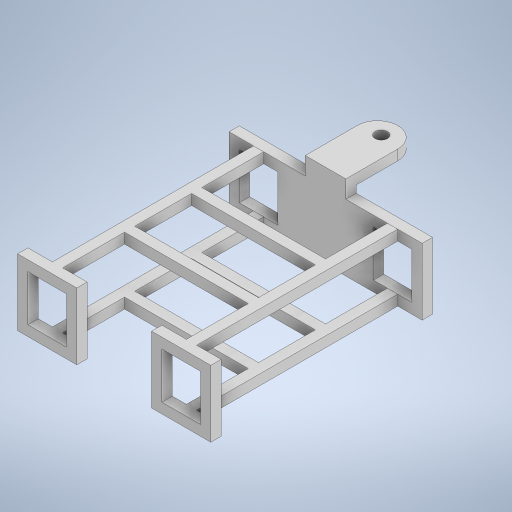
# Autodesk Inventor part: MHead
Saved by Autodesk Inventor 2024 (Build 280153000, 153)
## iProperties
Created: 2023-06-14
Part Number: MHead
Material: Generic
Document SubType Name: Modeling
Designer: vilas
Density: 1 g/cm^3
Appearance: Default
Author: vilas
Autodesk Inventor part; units mm, degrees
ref_plane "YZ Plane" through (0, 0, 0) normal (1, 0, 0) x (0, 1, 0)
sketch "Sketch1" plane through (0, 0, 0) normal (0, 0, 1) x (1, 0, 0)
  line L0 (-30, 11.15) -> (30, 11.15) construction
  line L1 (30, 11.15) -> (30, -11.15) construction
  line L2 (30, -11.15) -> (-30, -11.15) construction
  line L3 (-30, -11.15) -> (-30, 11.15) construction
  line L4 (-30, 11.15) -> (30, -11.15) construction
  line L5 (30, 11.15) -> (-30, -11.15) construction
  line L6 (-30, 11.15) -> (-35, 11.15)
  line L7 (-35, 11.15) -> (-35, 16.15)
  line L8 (-35, 16.15) -> (-30, 16.15)
  line L9 (-30, 16.15) -> (-30, 11.15)
  line L10 (30, 11.15) -> (35, 11.15)
  line L11 (35, 11.15) -> (35, 16.15)
  line L12 (35, 16.15) -> (30, 16.15)
  line L13 (30, 16.15) -> (30, 11.15)
  line L14 (30, -11.15) -> (35, -11.15)
  line L15 (35, -11.15) -> (35, -16.15)
  line L16 (35, -16.15) -> (30, -16.15)
  line L17 (30, -16.15) -> (30, -11.15)
  line L18 (-30, -11.15) -> (-35, -11.15)
  line L19 (-35, -11.15) -> (-35, -16.15)
  line L20 (-35, -16.15) -> (-30, -16.15)
  line L21 (-30, -16.15) -> (-30, -11.15)
  point P0 (0, 0)
  dimension "d0" = 60
  dimension "d1" = 22.3
  dimension "d2" = 5
  dimension "d3" = 5
  dimension "d4" = 5
  dimension "d5" = 5
  dimension "d6" = 5
  dimension "d7" = 5
  dimension "d8" = 5
  dimension "d9" = 5
  constraints: 44 end point, 10 parallel, 5 horizontal, 5 perpendicular, 2 midpoint
  measures "d0" distance of L1.end L2.end
  measures "d1" distance of L0.end L1.end
  measures "d2" distance of L7.end L8.end
  measures "d3" distance of L6.end L7.end
  measures "d4" distance of L12.end L11.end
  measures "d5" distance of L11.end L10.end
  measures "d6" distance of L15.end L16.end
  measures "d7" distance of L14.end L15.end
  measures "d8" distance of L20.end L19.end
  measures "d9" distance of L19.end L18.end
extrude "Extrusion1" add sketch "Sketch1" along normal mid plane 97.524
ref_plane "Work Plane1" through (0, 0, 48.762) normal (0, 0, 1) x (1, 0, 0)
sketch "Sketch2" plane through (0, 0, 48.762) normal (0, 0, 1) x (1, 0, 0)
  line L0 (0, 0) -> (-32.5, 0) construction
  line L1 (0, 0) -> (32.5, 0) construction
  line L2 (-46.85, 16.15) -> (-18.15, 16.15)
  line L3 (-18.15, 16.15) -> (-18.15, -16.15)
  line L4 (-18.15, -16.15) -> (-46.85, -16.15)
  line L5 (-46.85, -16.15) -> (-46.85, 16.15)
  line L6 (-46.85, 16.15) -> (-18.15, -16.15) construction
  line L7 (-18.15, 16.15) -> (-46.85, -16.15) construction
  line L8 (18.15, 16.15) -> (46.85, 16.15)
  line L9 (46.85, 16.15) -> (46.85, -16.15)
  line L10 (46.85, -16.15) -> (18.15, -16.15)
  line L11 (18.15, -16.15) -> (18.15, 16.15)
  line L12 (18.15, 16.15) -> (46.85, -16.15) construction
  line L13 (46.85, 16.15) -> (18.15, -16.15) construction
  line L14 (-23.15, 11.15) -> (-41.85, 11.15)
  line L15 (-41.85, 11.15) -> (-41.85, -11.15)
  line L16 (-41.85, -11.15) -> (-23.15, -11.15)
  line L17 (-23.15, -11.15) -> (-23.15, 11.15)
  line L18 (41.85, 11.15) -> (23.15, 11.15)
  line L19 (23.15, 11.15) -> (23.15, -11.15)
  line L20 (23.15, -11.15) -> (41.85, -11.15)
  line L21 (41.85, -11.15) -> (41.85, 11.15)
  dimension "d13" = 32.5
  dimension "d14" = 32.5
  dimension "d15" = 28.7
  dimension "d16" = 32.3
  dimension "d17" = 28.7
  dimension "d18" = 32.3
  dimension "d19" = 5
  dimension "d20" = 5
  constraints: 44 end point, 8 parallel, 4 horizontal, 4 midpoint, 4 perpendicular, 6 other
  measures "d13" distance of L0.start L0.end
  measures "d14" distance of L0.start L1.end
  measures "d15" distance of L3.end L4.end
  measures "d16" distance of L2.end L3.end
  measures "d17" distance of L9.end L10.end
  measures "d18" distance of L8.end L9.end
  measures "d19" distance between parallel lines of L2 L14
  measures "d20" distance between parallel lines of L8 L18
extrude "Extrusion2" add sketch "Sketch2" along normal blind 5
ref_plane "Work Plane2" through (0, 0, -48.771) normal (0, 0, 1) x (1, 0, 0)
sketch "Sketch4" plane through (0, 0, 0) normal (1, 0, 0) x (0, 1, 0)
  line L0 (11.15, -48.762) -> (11.15, 48.762) projected
  line L1 (11.15, 18.754) -> (16.15, 18.754)
  line L2 (16.15, 18.754) -> (16.15, 13.754)
  line L3 (16.15, 13.754) -> (11.15, 13.754)
  line L4 (11.15, 13.754) -> (11.15, 18.754)
  line L5 (-16.15, 48.762) -> (16.15, 48.762) projected
  line L6 (11.15, -13.754) -> (16.15, -13.754)
  line L7 (16.15, -13.754) -> (16.15, -18.754)
  line L8 (16.15, -18.754) -> (11.15, -18.754)
  line L9 (11.15, -18.754) -> (11.15, -13.754)
  line L10 (16.15, -48.762) -> (11.15, -48.762) projected
  line L11 (-11.15, 48.762) -> (-11.15, -48.762) projected
  line L12 (-11.15, 18.754) -> (-16.15, 18.754)
  line L13 (-16.15, 18.754) -> (-16.15, 13.754)
  line L14 (-16.15, 13.754) -> (-11.15, 13.754)
  line L15 (-11.15, 13.754) -> (-11.15, 18.754)
  line L16 (-11.15, -18.754) -> (-16.15, -18.754)
  line L17 (-16.15, -18.754) -> (-16.15, -13.754)
  line L18 (-16.15, -13.754) -> (-11.15, -13.754)
  line L19 (-11.15, -13.754) -> (-11.15, -18.754)
  line L20 (-11.15, -48.762) -> (-16.15, -48.762) projected
  point P0 (0, 0)
  dimension "d30" = 5
  dimension "d31" = 5
  dimension "d32" = 30.008
  dimension "d33" = 5
  dimension "d34" = 5
  dimension "d35" = 30.008
  dimension "d36" = 5
  dimension "d37" = 5
  dimension "d38" = 5
  dimension "d39" = 5
  dimension "d40" = 30.008
  dimension "d41" = 30.008
  constraints: 32 end point, 8 parallel, 4 horizontal, 4 perpendicular, 4 point on line
  measures "d30" distance of L2.end L3.end
  measures "d31" distance of L1.end L2.end
  measures "d32" distance between parallel lines of L1 L5
  measures "d33" distance of L7.end L8.end
  measures "d34" distance of L6.end L7.end
  measures "d35" distance between parallel lines of L8 L10
  measures "d36" distance of L14.end L13.end
  measures "d37" distance of L13.end L12.end
  measures "d38" distance of L17.end L18.end
  measures "d39" distance of L16.end L17.end
  measures "d40" distance between parallel lines of L16 L20
  measures "d41" distance between parallel lines of L12 L5
extrude "Extrusion4" add sketch "Sketch4" along normal mid plane 60
sketch "Sketch7" plane through (0, 0, -48.771) normal (0, 0, 1) x (1, 0, 0)
  line L0 (-46.85, -16.15) -> (-18.15, -16.15) projected
  line L1 (46.85, 16.15) -> (-46.85, 16.15)
  line L2 (-46.85, 16.15) -> (-46.85, -16.15)
  line L3 (-46.85, -16.15) -> (46.85, -16.15)
  line L4 (46.85, -16.15) -> (46.85, 16.15)
  line L5 (46.85, 16.15) -> (-46.85, -16.15) construction
  line L6 (-46.85, 16.15) -> (46.85, -16.15) construction
  line L7 (0, 0) -> (32.5, 0) construction
  line L8 (0, 0) -> (-32.5, 0) construction
  line L9 (41.85, -11.15) -> (23.15, -11.15) projected
  line L10 (23.15, 11.15) -> (41.85, 11.15)
  line L11 (41.85, 11.15) -> (41.85, -11.15)
  line L12 (41.85, -11.15) -> (23.15, -11.15)
  line L13 (23.15, -11.15) -> (23.15, 11.15)
  line L14 (23.15, 11.15) -> (41.85, -11.15) construction
  line L15 (41.85, 11.15) -> (23.15, -11.15) construction
  line L16 (-41.85, -11.15) -> (-41.85, 11.15) projected
  line L17 (-23.15, 11.15) -> (-41.85, 11.15)
  line L18 (-41.85, 11.15) -> (-41.85, -11.15)
  line L19 (-41.85, -11.15) -> (-23.15, -11.15)
  line L20 (-23.15, -11.15) -> (-23.15, 11.15)
  line L21 (-23.15, 11.15) -> (-41.85, -11.15) construction
  line L22 (-41.85, 11.15) -> (-23.15, -11.15) construction
  line L23 (0, 0) -> (0, 24.693) construction
  line L24 (0, 24.693) -> (9.85, 24.693) construction
  line L25 (9.85, 24.693) -> (-9.85, 24.693)
  line L26 (-9.85, 24.693) -> (-9.85, 16.15)
  line L27 (-9.85, 16.15) -> (9.85, 16.15)
  line L28 (9.85, 16.15) -> (9.85, 24.693)
  dimension "d61" = 32.5
  dimension "d62" = 32.5
  dimension "d63" = 24.693
  dimension "d64" = 9.85
  dimension "d65" = 19.7
  constraints: 52 end point, 8 parallel, 6 horizontal, 6 midpoint, 5 perpendicular, 1 point on line, 1 vertical
  measures "d61" distance of L7.start L7.end
  measures "d62" distance of L7.start L8.end
  measures "d63" distance of L7.start L23.end
  measures "d64" distance of L23.end L24.end
  measures "d65" distance of L27.end L26.end
extrude "Extrusion7" add sketch "Sketch7" against normal blind 5
sketch "Sketch8" plane through (0, 0, -53.771) normal (0, 0, -1) x (-1, 0, 0)
  line L0 (9.85, 24.693) -> (-9.85, 24.693) projected
  line L1 (9.85, 16.15) -> (9.85, 24.693) projected
  line L2 (-9.85, 24.693) -> (9.85, 24.693)
  line L3 (9.85, 24.693) -> (9.85, 19.693)
  line L4 (9.85, 19.693) -> (-9.85, 19.693)
  line L5 (-9.85, 19.693) -> (-9.85, 24.693)
  point P0 (0, 0)
  dimension "d68" = 5
  constraints: 8 end point, 2 parallel, 1 horizontal, 1 perpendicular, 1 point on line
  measures "d68" distance of L2.end L3.end
extrude "Extrusion8" add sketch "Sketch8" along normal blind 30
fillet "Fillet2" radius 9.85 2 edges at (9.85, 22.193, -83.771) (-9.85, 22.193, -83.771)
sketch "Sketch9" plane through (-9.85, 19.693, -53.771) normal (0, -1, 0) x (1, 0, 0)
  line L0 (56.7, 0) -> (-37, 0) projected
  line L1 (9.85, 0) -> (9.85, -30) construction
  arc A0 (0, -20.15) -> (19.7, -20.15) centre (9.85, -20.15) ccw projected
  circle A1 centre (9.85, -22) radius 3
  point P0 (9.85, 53.771)
  dimension "d72" = 6
  dimension "d73" = 22
  constraints: 2 end point, 1 centre point, 1 midpoint, 1 point on circle, 1 point on line, 1 vertical
  measures "d72" diameter of A1
  measures "d73" distance from line of L0 A1.centre
extrude "Extrusion9" cut sketch "Sketch9" against normal through all
body "Solid1"
